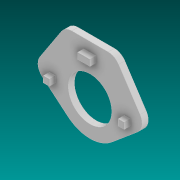
# Autodesk Inventor part: lager opvulling voor lijm
Saved by Autodesk Inventor 2020 (Build 240168000, 168)
## iProperties
Created: 2020-05-27
Part Number: lager opvulling voor lijm
Material: Generic
Document SubType Name: Modeling
Designer: stefa
Density: 1 g/cm^3
Appearance: Default
Author: stefa
Autodesk Inventor part; units mm, degrees
ref_plane "YZ Plane" through (0, 0, 0) normal (1, 0, 0) x (0, 1, 0)
ref_plane "XZ Plane" through (0, 0, 0) normal (0, 1, 0) x (-1, 0, 0)
ref_plane "XY Plane" through (0, 0, 0) normal (0, 0, 1) x (1, 0, 0)
sketch "Sketch1" plane through (0, 0, 0) normal (0, 0, 1) x (1, 0, 0)
  circle A0 centre (0, 0) radius 7
  circle A1 centre (0, 0) radius 11
  line L0 (-31.215, 0) -> (-15, 0) construction
  line L1 (-11.7494, 0) -> (27.9854, 0) construction
  line L2 (7.0707, -8.4265) -> (18, 0.7443)
  line L3 (18, 0.7443) -> (8, 16)
  line L4 (8, 16) -> (0, 16)
  line L5 (0, -17.2006) -> (0, 31.2913) construction
  line L6 (-7.0707, -8.4265) -> (-18, 0.7443)
  line L7 (-18, 0.7443) -> (-8, 16)
  line L8 (-8, 16) -> (0, 16)
  dimension "d12" = 22
  dimension "d11" = 14
  dimension "d13" = 50
  dimension "d14" = 18
  dimension "d15" = 16
  dimension "d16" = 8
  constraints: 18 end point, 3 symmetric about line, 2 coincident, 2 horizontal, 2 point on line, 1 centre point, 1 parallel, 1 vertical, 4 other
  measures "d11" diameter of A0
  measures "d13" angle of L5 L2
  measures "d14" distance from line of L5 L2.end
  measures "d15" distance from line of A0.centre L4
  measures "d16" distance from line of L5 L3.end
extrude "Extrusion1" add sketch "Sketch1" along normal blind 2
sketch "Sketch2" plane through (0, 0, 2) normal (0, 0, 1) x (1, 0, 0)
  arc A0 (-7.0707, -8.4265) -> (7.0707, -8.4265) centre (0, 0) ccw projected
  line L0 (7.0707, -8.4265) -> (18, 0.7443) projected
  line L1 (18, 0.7443) -> (8, 16) projected
  line L2 (8, 16) -> (-8, 16) projected
  line L3 (-8, 16) -> (-18, 0.7443) projected
  line L4 (-18, 0.7443) -> (-7.0707, -8.4265) projected
  circle A1 centre (0, 0) radius 7 projected
  line L5 (11, -1) -> (13, -1)
  line L6 (13, -1) -> (13, 1)
  line L7 (13, 1) -> (11, 1)
  line L8 (11, 1) -> (11, -1)
  line L9 (11, -1) -> (13, 1) construction
  line L10 (13, -1) -> (11, 1) construction
  line L11 (-2, 13) -> (2, 13)
  line L12 (2, 13) -> (2, 11)
  line L13 (2, 11) -> (-2, 11)
  line L14 (-2, 11) -> (-2, 13)
  line L15 (-2, 13) -> (2, 11) construction
  line L16 (2, 13) -> (-2, 11) construction
  line L17 (0, 16) -> (0, -7) construction
  line L18 (-11, -1) -> (-13, -1)
  line L19 (-13, -1) -> (-13, 1)
  line L20 (-13, 1) -> (-11, 1)
  line L21 (-11, 1) -> (-11, -1)
  line L22 (-11, -1) -> (-13, 1) construction
  line L23 (-13, -1) -> (-11, 1) construction
  point P0 (12, 0)
  point P1 (0, 12)
  point P2 (12, 0)
  point P3 (0, 12)
  point P4 (0, 12)
  point P5 (-12, 0)
  point P6 (-12, 0)
  dimension "d18" = 2
  dimension "d19" = 2
  dimension "d20" = 4
  dimension "d21" = 2
  dimension "d22" = 12
  dimension "d23" = 12
  constraints: 38 end point, 10 midpoint, 6 symmetric about line, 4 parallel, 2 horizontal, 2 perpendicular, 2 vertical alignment, 1 horizontal alignment, 1 vertical, 1 other
  measures "d18" distance of L7.end L6.end
  measures "d19" distance of L6.end L5.end
  measures "d20" distance of L12.end L13.end
  measures "d21" distance of L11.end L12.end
  measures "d22" distance of point (0, 0) point (0, 12)
  measures "d23" distance of point (0, 0) point (12, 0)
extrude "Extrusion2" add sketch "Sketch2" along normal blind 2 contours L8 L7 L6 L5 | L11 L12 L13 L14 | L18 L19 L20 L21
fillet "Fillet1" radius 4 4 edges at (18, 0.7443, 1) (-18, 0.7443, 1) (-8, 16, 1) (8, 16, 1)
body "Solid1"
